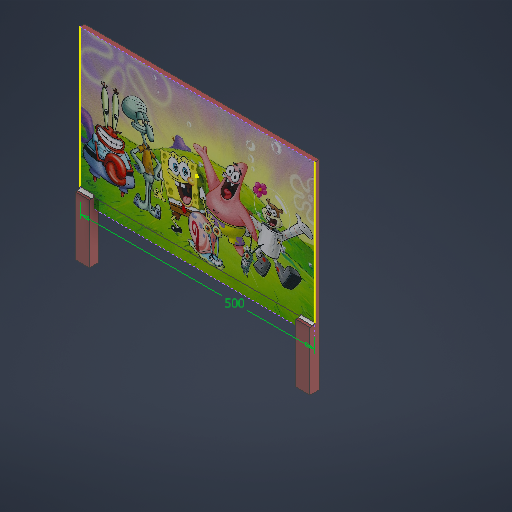
# Autodesk Inventor part: Stand of theme
Saved by Autodesk Inventor 2026.2 (Build 302298010, 298A)
## iProperties
Created: 2026-05-30
Part Number: Stand of theme
Material: Generic
Document SubType Name: Modeling
Designer: lenovo
Density: 1 g/cm^3
Appearance: Default
Author: lenovo
Autodesk Inventor part; units mm, degrees
ref_plane "YZ Plane" through (0, 0, 0) normal (1, 0, 0) x (0, 1, 0)
ref_plane "XZ Plane" through (0, 0, 0) normal (0, 1, 0) x (-1, 0, 0)
ref_plane "XY Plane" through (0, 0, 0) normal (0, 0, 1) x (1, 0, 0)
sketch "Sketch1" plane through (0, 0, 0) normal (0, 0, 1) x (1, 0, 0)
  line L0 (-250, -150) -> (250, -150)
  line L1 (250, -150) -> (250, 150)
  line L2 (250, 150) -> (-250, 150)
  line L3 (-250, 150) -> (-250, -150)
  line L4 (-250, -150) -> (250, 150) construction
  line L5 (250, -150) -> (-250, 150) construction
  line L6 (-250, -150) -> (-250, -275)
  line L7 (-250, -275) -> (-220, -275)
  line L8 (-220, -275) -> (-220, -150)
  line L9 (250, -150) -> (250, -275)
  line L10 (250, -275) -> (220, -275)
  line L11 (220, -275) -> (220, -150)
  point P0 (0, 0)
  dimension "d0" = 500
  dimension "d1" = 300
  dimension "d4" = 30
  dimension "d5" = 30
  dimension "d15" = 125
  constraints: 24 end point, 5 perpendicular, 4 point on line, 2 midpoint, 2 parallel, 1 horizontal, 1 vertical
  measures "d0" distance of L2.end L1.end
  measures "d1" distance of L1.end L0.end
  measures "d4" distance of L6.end L7.end
  measures "d5" distance of L9.end L10.end
  measures "d15" distance of L0.start L6.end
extrude "Extrusion1" add sketch "Sketch1" along normal blind 10 contours L3 L2 L1 L0
extrude "Extrusion2" add sketch "Sketch1" along normal blind 20 contours L0 L8 L7 L6 | L0 L9 L10 L11
fillet "Face Fillet1" radius 4.13 1 edges at (235, -150, 10)
fillet "Face Fillet2" radius 5.05 1 edges at (-235, -150, 10)
sketch "Sketch4" plane through (0, 0, 10) normal (0, 0, 1) x (1, 0, 0)
  line L0 (-250, 150) -> (-250, -144.95) projected
  line L1 (-250, 150) -> (250, 150) construction
  line L2 (250, 150) -> (250, -171.25) construction
  line L3 (250, -171.25) -> (-250, -171.25) construction
  line L4 (-250, -171.25) -> (-250, 150) construction
  line L5 (250, -145.87) -> (250, 150) projected
  point P0 (0, 0)
  dimension "d97" = 500
  constraints: 2 other
  measures "d97" distance of L2.end L3.end
body "Solid1"
